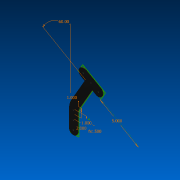
# Autodesk Inventor part: Hood Upper Bracket
Saved by Autodesk Inventor 2022.2 (Build 262287000, 287)
## iProperties
Created: 2022-04-17
Part Number: Hood Upper Bracket
Material: PET Plastic
Document SubType Name: Modeling
Designer: omard
Density: 1.541 g/cm^3
Appearance: Smooth - Black
Author: omard
Autodesk Inventor part; units mm, degrees
ref_plane "YZ Plane" through (0, 0, 0) normal (1, 0, 0) x (0, 1, 0)
ref_plane "XZ Plane" through (0, 0, 0) normal (0, 1, 0) x (-1, 0, 0)
ref_plane "XY Plane" through (0, 0, 0) normal (0, 0, 1) x (1, 0, 0)
sketch "Sketch1" plane through (0, 0, 0) normal (0, 0, 1) x (1, 0, 0)
  line L0 (-12.7, 25.4) -> (12.7, 25.4)
  line L1 (12.7, 25.4) -> (12.7, -25.4)
  line L2 (12.7, -25.4) -> (-12.7, -25.4)
  line L3 (-12.7, -25.4) -> (-12.7, 25.4)
  line L4 (-12.7, 25.4) -> (12.7, -25.4) construction
  line L5 (12.7, 25.4) -> (-12.7, -25.4) construction
  line L6 (45.5925, 124.1219) -> (89.5866, 98.7219)
  line L7 (89.5866, 98.7219) -> (76.8866, 76.7248)
  line L8 (76.8866, 76.7248) -> (32.8925, 102.1248)
  line L9 (32.8925, 102.1248) -> (45.5925, 124.1219)
  line L10 (45.5925, 124.1219) -> (76.8866, 76.7248) construction
  line L11 (89.5866, 98.7219) -> (32.8925, 102.1248) construction
  line L12 (50.2411, 106.7734) -> (72.2381, 94.0734) construction
  line L13 (0, -12.7) -> (0, 12.7) construction
  line L14 (-12.7, -25.4) -> (12.7, -25.4)
  line L15 (12.7, -25.4) -> (12.7, -50.8)
  line L16 (12.7, -50.8) -> (-12.7, -50.8)
  line L17 (-12.7, -50.8) -> (-12.7, -25.4)
  circle A0 centre (0, -38.1) radius 12.7
  line L18 (54.8896, 89.4248) -> (32.8925, 102.1248)
  line L19 (32.8925, 102.1248) -> (-5.3784, 35.8376)
  line L20 (-5.3784, 35.8376) -> (16.6186, 23.1376)
  line L21 (16.6186, 23.1376) -> (54.8896, 89.4248)
  line L22 (186.8719, 13.2248) -> (-11.1015, 127.5248) construction
  line L23 (45.5925, 124.1219) -> (32.8925, 102.1248)
  line L24 (32.8925, 102.1248) -> (10.8955, 114.8248)
  line L25 (10.8955, 114.8248) -> (23.5955, 136.8219)
  line L26 (23.5955, 136.8219) -> (45.5925, 124.1219)
  line L27 (28.244, 119.4734) -> (50.2411, 106.7734) construction
  arc A1 (-5.3784, 35.8376) -> (-12.7, 8.5131) centre (41.949, 8.5131) ccw
  arc A2 (16.6186, 23.1376) -> (12.7, 8.5131) centre (41.949, 8.5131) ccw
  arc A3 (34.594, 130.4719) -> (21.894, 108.4748) centre (28.244, 119.4734) ccw
  circle A4 centre (72.2381, 94.0734) radius 12.7
  point P0 (0, 0)
  point P1 (0, 0)
  point P2 (0, 0)
  point P3 (61.2396, 100.4234)
  point P4 (61.2396, 100.4234)
  point P5 (-12.7, -38.1)
  point P6 (12.7, -38.1)
  point P7 (65.8881, 83.0748)
  point P8 (78.5881, 105.0719)
  dimension "d0" = 25.4
  dimension "d1" = 50.8
  dimension "d2" = 25.4
  dimension "d3" = 12.7
  dimension "d6" = 60
  dimension "d14" = 127
  constraints: 56 end point, 11 parallel, 10 midpoint, 8 tangent, 7 equal length, 6 collinear, 6 point on circle, 5 centre point, 5 perpendicular, 4 point on line, 3 coincident, 2 horizontal, 2 vertical alignment, 1 vertical, 3 other
  measures "d0" distance between parallel lines of L3 L1
  measures "d1" distance between parallel lines of L2 L0
  measures "d2" distance of L13.start L13.end
  measures "d3" distance of L13.start point (0, 0)
  measures "d6" angle of L3 L8
  measures "d14" distance of L22.start L7.end
extrude "Extrusion1" add sketch "Sketch1" along normal blind 3.175 contours A1 L20 L0 | L0 L1 L2 L3 A1 | L20 A2 L1 | L20 L19 L8 L21 | L2 A0 L17 | L9 L6 A4 L8 | L24 A3 L26 L9 | L2 L15 A0 | A0 | A4
hole "Hole1" at (0, -12.7, 0) at (0, 12.7, 0) at (72.2381, 94.0734, 0) at (50.2411, 106.7734, 0) at (0, -38.1, 0) at (28.244, 119.4734, 0) direction (0, 0, 1) diameter 4.445 end through all start extended yes
fillet "Fillet1" radius 12.7 2 edges at (32.8925, 102.1248, 1.5875) (54.8896, 89.4248, 1.5875)
equation "\"d3\" = 0.5 * d2"
body "Solid1"
